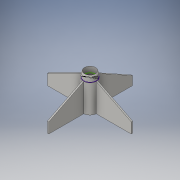
# Autodesk Inventor part: Rocket - Base Assembled
Saved by Autodesk Inventor 2016 (Build 200138000, 138)
## iProperties
Created: 2015-06-23
Part Number: Rocket - Base Assembled
Material: Generic
Document SubType Name: Modeling
Designer: The Shack
Density: 1 g/cm^3
Appearance: Default
Author: The Shack
Autodesk Inventor part; units mm, degrees
ref_plane "YZ Plane" through (0, 0, 0) normal (1, 0, 0) x (0, 1, 0)
ref_plane "XZ Plane" through (0, 0, 0) normal (0, 1, 0) x (-1, 0, 0)
ref_plane "XY Plane" through (0, 0, 0) normal (0, 0, 1) x (1, 0, 0)
sketch "Sketch1" plane through (0, 0, 0) normal (0, 1, 0) x (-1, 0, 0)
  circle A0 centre (0, 0) radius 6.35
  dimension "d0" = 12.7
  constraints: 1 centre point, 1 coincident
  measures "d0" diameter of A0
extrude "Extrusion1" add sketch "Sketch1" along normal blind 25.4
sketch "Sketch2" plane through (0, 25.4, 0) normal (0, 1, 0) x (1, 0, 0)
  circle A0 centre (0, 0) radius 5.715
  circle A1 centre (0, 0) radius 5.0201
  dimension "d3" = 11.43
  constraints: 2 centre point, 2 coincident
  measures "d3" diameter of A0
extrude "Extrusion2" cut sketch "Sketch2" against normal blind 25.4 contours A1
extrude "Extrusion3" add sketch "Sketch2" along normal blind 5.08
fillet "Fillet1" radius 2.54 1 edges at (-5.715, 30.48, 0)
sketch "Sketch3" plane through (0, 0, 0) normal (0, 1, 0) x (-1, 0, 0)
  point P0 (0, 0)
sketch "Sketch4" plane through (0, 0, 0) normal (0, 0, 1) x (1, 0, 0)
  line L0 (-6.35, 0) -> (6.35, 0) projected
  line L1 (6.35, 0) -> (38.1, 0)
  line L2 (-6.35, 0) -> (-38.1, 0)
  line L3 (-38.1, 0) -> (-38.1, 9.525)
  line L4 (6.35, 25.4) -> (-6.35, 25.4) projected
  line L5 (-38.1, 9.525) -> (-6.35, 25.4)
  line L6 (-6.35, 25.4) -> (-6.35, 0)
  line L7 (6.35, 25.4) -> (6.35, 0)
  line L8 (6.35, 25.4) -> (38.1, 9.525)
  line L9 (38.1, 9.525) -> (38.1, 0)
  point P0 (0, 0)
  dimension "d9" = 31.75
  dimension "d10" = 31.75
  constraints: 16 end point, 2 horizontal, 2 parallel, 2 perpendicular
  measures "d9" distance of L0.end L1.end
  measures "d10" distance of L0.start L2.end
extrude "Extrusion4" add sketch "Sketch4" along normal mid plane 1.27 contours L2 L3 L5 L6 | L7 L8 L9 L1
sketch "Sketch5" plane through (0, 0, 0) normal (1, 0, 0) x (0, 1, 0)
  line L0 (0, -6.35) -> (0, -38.1)
  line L1 (0, -38.1) -> (7.7611, -38.1)
  line L2 (25.4, -6.35) -> (25.4, 0) projected
  line L3 (7.7611, -38.1) -> (25.4, -6.35)
  line L4 (25.4, -6.35) -> (0, -6.35)
  line L5 (0, -6.35) -> (25.4, -6.35) projected
  line L6 (0, 6.35) -> (0, 38.1)
  line L7 (0, 38.1) -> (9.525, 38.1)
  line L8 (25.4, 0) -> (25.4, 6.35) projected
  line L9 (9.525, 38.1) -> (25.4, 6.35)
  line L10 (25.4, 6.35) -> (0, 6.35)
  point P0 (0, 0)
  dimension "d15" = 31.75
  dimension "d16" = 31.75
  constraints: 16 end point, 3 perpendicular, 1 collinear, 1 point on line, 1 vertical
  measures "d15" distance from line of L4 L0.end
  measures "d16" distance between parallel lines of L7 L10
extrude "Extrusion5" add sketch "Sketch5" along normal mid plane 1.27
sketch "Sketch6" plane through (0, 0, 0) normal (0, -1, 0) x (1, 0, 0)
  circle A0 centre (0, 0) radius 5.0201 projected
  line L0 (-4.9798, 0.635) -> (-1.8048, 0.635)
  line L1 (-6.35, 0.635) -> (-38.1, 0.635) projected
  line L2 (-1.8048, 0.635) -> (-1.8048, -0.889)
  line L3 (-1.8048, -0.889) -> (-4.9408, -0.889)
  spline S0 degree 1 poles (-4.9798, 0.635) (-4.9408, -0.889) knots 0 0 1 1
  line L4 (4.9408, 0.889) -> (1.7658, 0.889)
  line L5 (1.7658, 0.889) -> (1.7658, -0.889)
  line L6 (1.7658, -0.889) -> (4.9408, -0.889)
  line L7 (4.9408, 0.889) -> (4.9408, -0.889)
  dimension "d17" = 3.175
  dimension "d18" = 1.524
  dimension "d19" = 3.175
  constraints: 14 end point, 4 perpendicular, 4 point on circle, 1 collinear, 1 horizontal, 1 vertical, 2 other
  measures "d17" distance of L0.start L0.end
  measures "d18" distance of L0.end L2.end
  measures "d19" distance of L4.start L4.end
extrude "Extrusion6" add sketch "Sketch6" against normal blind 2.54 contours L7 L6 L5 L4 | L0 L2 L3 S0
body "Solid1"
